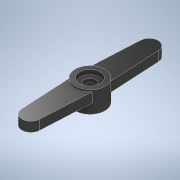
# Autodesk Inventor part: attachmnet
Saved by Autodesk Inventor 2022 (Build 260153000, 153)
## iProperties
Created: 2022-02-11
Part Number: attachmnet
Material: Nylon 6/6
Document SubType Name: Modeling
Designer: juanp
Density: 1.13 g/cm^3
Appearance: Nylon 6
Author: juanp
Autodesk Inventor part; units mm, degrees
ref_plane "YZ Plane" through (0, 0, 0) normal (1, 0, 0) x (0, 1, 0)
ref_plane "XZ Plane" through (0, 0, 0) normal (0, 1, 0) x (-1, 0, 0)
ref_plane "XY Plane" through (0, 0, 0) normal (0, 0, 1) x (1, 0, 0)
sketch "Sketch1" plane through (0, 0, 0) normal (0, 1, 0) x (-1, 0, 0)
  circle A0 centre (0, 0) radius 3.35
  dimension "d0" = 6.7
  constraints: 1 centre point, 1 coincident
  measures "d0" diameter of A0
extrude "Extrusion1" add sketch "Sketch1" along normal blind 4.8
ref_plane "Work Plane1" through (0, 4.4, 0) normal (0, 1, 0) x (1, 0, 0)
sketch "Sketch2" plane through (0, 4.4, 0) normal (0, 1, 0) x (1, 0, 0)
  circle A0 centre (0, 0) radius 3.35 projected
  line L0 (-2.6, 2.1125) -> (-2, 13.453)
  circle A1 centre (0, 0) radius 3.35 projected
  line L1 (2.6, 2.1125) -> (2, 13.453)
  arc A2 (2, 13.453) -> (-2, 13.453) centre (0, 13.3472) ccw
  line L2 (-2, 13.453) -> (2, 13.453) construction
  line L3 (2.6, 2.1125) -> (-2.6, 2.1125) construction
  line L4 (0, 0) -> (-1.2831, 0)
  line L5 (-2.6, -2.1125) -> (-2, -13.453)
  line L6 (2.6, -2.1125) -> (2, -13.453)
  arc A3 (-2, -13.453) -> (2, -13.453) centre (0, -13.3472) ccw
  line L7 (-2, -13.453) -> (2, -13.453) construction
  line L8 (2.6, -2.1125) -> (-2.6, -2.1125) construction
  dimension "d4" = 5.2
  dimension "d5" = 12
  dimension "d6" = 4
  constraints: 18 end point, 5 point on circle, 5 symmetric about line, 3 horizontal, 2 centre point, 2 tangent, 3 other
  measures "d4" distance of L1.start L0.start
  measures "d6" distance of L0.end L1.end
extrude "Extrusion2" add sketch "Sketch2" against normal blind 2.2 contours A0 L0 A2 L1 | L6 A3 L5 A0
sketch "Sketch3" plane through (0, 4.8, 0) normal (0, 1, 0) x (1, 0, 0)
  circle A0 centre (0, 0) radius 1.25
  circle A1 centre (0, 0) radius 2.3
  dimension "d9" = 2.5
  dimension "d10" = 4.6
  constraints: 2 centre point, 2 coincident
  measures "d9" diameter of A0
  measures "d10" diameter of A1
extrude "Extrusion3" cut sketch "Sketch3" against normal through all contours A0
extrude "Extrusion4" cut sketch "Sketch3" against normal blind 1
sketch "Sketch4" plane through (0, 0, 0) normal (0, -1, 0) x (1, 0, 0)
  circle A0 centre (0, 0) radius 2.35
  dimension "d15" = 4.7
  constraints: 1 centre point, 1 coincident
  measures "d15" diameter of A0
extrude "Extrusion5" cut sketch "Sketch4" against normal blind 2.9
body "Solid1"
